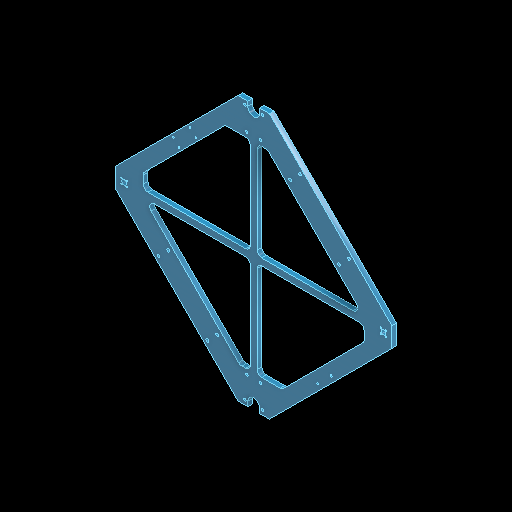
# Autodesk Inventor part: z_plate
Saved by Autodesk Inventor 2026.1 (Build 301233000, 233)
## iProperties
Created: 2025-09-21
Part Number: z_plate
Material: Aluminum 6061
Document SubType Name: Modeling
Designer: drago
Density: 2.7 g/cm^3
Appearance: Sky Blue Dark
Mass: 2273.65 g
Surface Area: 2214.69 cm^2
Volume: 842.092 cm^3
Author: drago
Autodesk Inventor part; units mm, degrees
ref_plane "YZ Plane" through (0, 0, 0) normal (1, 0, 0) x (0, 1, 0)
ref_plane "XZ Plane" through (0, 0, 0) normal (0, 1, 0) x (-1, 0, 0)
sketch "Sketch2" plane through (0, 0, 0) normal (0, 0, 1) x (1, 0, 0)
  circle A0 centre (0, 277.5) radius 8 construction
  circle A1 centre (0, 277.5) radius 13
  circle A2 centre (0, 277.5) radius 10.5 construction
  line L0 (25, 287.5) -> (-25, 287.5) construction
  line L1 (-25, 287.5) -> (-25, 222.5) construction
  line L2 (-25, 222.5) -> (25, 222.5) construction
  line L3 (25, 222.5) -> (25, 287.5) construction
  circle A3 centre (15, 228.5) radius 2.7
  circle A4 centre (-15, 228.5) radius 2.7
  circle A5 centre (-19, 277.5) radius 2.7
  circle A6 centre (19, 277.5) radius 2.7
  circle A7 centre (0, -277.5) radius 8 construction
  circle A8 centre (0, -277.5) radius 13
  circle A9 centre (0, -277.5) radius 10.5 construction
  line L4 (25, -287.5) -> (-25, -287.5) construction
  line L5 (-25, -287.5) -> (-25, -222.5) construction
  line L6 (-25, -222.5) -> (25, -222.5) construction
  line L7 (25, -222.5) -> (25, -287.5) construction
  circle A10 centre (-15, -228.5) radius 2.7
  circle A11 centre (15, -228.5) radius 2.7
  circle A12 centre (-19, -277.5) radius 2.7
  circle A13 centre (19, -277.5) radius 2.7
  line L8 (10.5, -277.5) -> (10.5, -287.5) construction
  line L9 (-10.5, -277.5) -> (-10.5, -287.5) construction
  line L10 (10.5, 277.5) -> (10.5, 287.5) construction
  line L11 (-10.5, 277.5) -> (-10.5, 287.5) construction
  circle A14 centre (281.7, 0) radius 5.25
  circle A15 centre (-281.7, 0) radius 5.25
  line L12 (0, -321.7336) -> (321.7336, 0)
  line L13 (321.7336, 0) -> (0, 321.7336)
  line L14 (0, 321.7336) -> (-321.7336, 0)
  line L15 (-321.7336, 0) -> (0, -321.7336)
  line L16 (321.7336, 0) -> (-321.7336, 0) construction
  line L17 (0, -321.7336) -> (455, -321.7336) construction
  line L18 (300.5, 21.2336) -> (300.5, -21.2336)
  line L19 (-300.5, 21.2336) -> (-300.5, -21.2336)
  line L20 (-24.2336, 297.5) -> (24.2336, 297.5) construction
  line L21 (-34.2336, 287.5) -> (34.2336, 287.5)
  line L22 (-24.2336, -297.5) -> (24.2336, -297.5) construction
  line L23 (-34.2336, -287.5) -> (34.2336, -287.5)
  line L24 (-9.5, 297.5) -> (-3.976, 284.442) construction
  line L25 (9.5, 297.5) -> (3.976, 284.442) construction
  line L26 (-14.929, 297.5) -> (-9.9883, 285.8207)
  line L27 (14.929, 297.5) -> (9.9883, 285.8207)
  line L28 (-9.5, -297.5) -> (-3.976, -284.442) construction
  line L29 (9.5, -297.5) -> (3.976, -284.442) construction
  line L30 (14.929, -297.5) -> (9.9883, -285.8207)
  line L31 (-14.929, -297.5) -> (-9.9883, -285.8207)
  line L32 (13, 277.5) -> (13, 287.5)
  line L33 (-13, 277.5) -> (-13, 287.5)
  line L34 (-13, -277.5) -> (-13, -287.5)
  line L35 (13, -277.5) -> (13, -287.5)
  line L36 (281.7, 0) -> (287.3569, 5.6569) construction
  line L37 (281.7, 0) -> (289.7, 0) construction
  circle A16 centre (287.3569, 5.6569) radius 1.6
  circle A17 centre (276.0431, 5.6569) radius 1.6
  circle A18 centre (276.0431, -5.6569) radius 1.6
  circle A19 centre (287.3569, -5.6569) radius 1.6
  line L38 (-281.7, 0) -> (-287.3569, 5.6569) construction
  circle A20 centre (-287.3569, 5.6569) radius 1.6
  circle A21 centre (-287.3569, -5.6569) radius 1.6
  circle A22 centre (-276.0431, -5.6569) radius 1.6
  circle A23 centre (-276.0431, 5.6569) radius 1.6
  line L39 (0, -321.7336) -> (0, 321.7336) construction
  point P0 (0, 0)
  point P1 (-10.6987, -287.5)
  point P2 (10.6987, -287.5)
  point P3 (10.6987, 287.5)
  point P4 (-10.6987, 287.5)
  point P5 (300.5, 292.5)
  point P6 (300.5, -292.5)
  point P7 (-300.5, -292.5)
  point P8 (-300.5, 292.5)
  dimension "d256" = 16
  dimension "d258" = 277.5
  dimension "d259" = 26
  dimension "d260" = 21
  dimension "d262" = 10
  dimension "d263" = 65
  dimension "d271" = 6
  dimension "d272" = 10
  dimension "d275" = 6
  dimension "d276" = 10
  dimension "d285" = 10
  dimension "d300" = 10.5
  dimension "d302" = 281.7
  dimension "d321" = 45
  dimension "d322" = 455
  dimension "d323" = 18.8
  dimension "d325" = 20
  dimension "d330" = 67.07
  dimension "d331" = 9.5
  dimension "d336" = 14.929
  dimension "d391" = 8
  dimension "d392" = 45
  dimension "d394" = 3.2
  dimension "d397" = 360
  dimension "d399" = 8
  dimension "d400" = 45
  dimension "d404" = 360
  dimension "d432" = 5.4
  dimension "d433" = 50
  dimension "d483" = 10
  constraints: 80 end point, 34 point on line, 24 centre point, 16 point on circle, 12 equal radius, 9 perpendicular, 8 equal length, 8 symmetric about line, 7 horizontal, 6 coincident, 6 parallel, 6 tangent, 5 vertical, 2 midpoint, 27 other
  measures "d256" diameter of A0
  measures "d258" distance of point (0, 0) A0.centre
  measures "d259" diameter of A1
  measures "d260" diameter of A2
  measures "d262" distance from line of A2.centre L0
  measures "d263" distance of L0.end L1.end
  measures "d271" distance from line of L2 A3.centre
  measures "d272" distance from line of L3 A3.centre
  measures "d275" distance from line of L3 A6.centre
  measures "d276" distance from line of L0 A6.centre
  measures "d285" distance from line of L4 A8.centre
  measures "d300" diameter of A14
  measures "d302" distance of point (0, 0) L36.start
  measures "d321" angle of L17 L12
  measures "d322" distance of L13.end L12.end
  measures "d323" distance from line of L18 L36.start
  measures "d325" distance from line of A1.centre L20
  measures "d330" angle of L25 L20
  measures "d331" horizontal distance of A1.centre L25.start
  measures "d336" horizontal distance of A1.centre L27.start
  measures "d391" distance of L36.start L36.end
  measures "d392" angle of L37 L36
  measures "d394" diameter of A16
  measures "d399" distance of L38.start L38.end
  measures "d400" angle of L16 L38
  measures "d432" diameter of A3
  measures "d433" distance of L1.end L2.end
  measures "d483" distance from line of A1.centre L21
ref_plane "Work Plane1" through (0, 0, 0) normal (0, 0, 1) x (1, 0, 0)
sketch "Sketch3" plane through (0, 0, 0) normal (0, 0, 1) x (1, 0, 0)
  line L0 (-160.8668, -160.8668) -> (160.8668, 160.8668) construction
  line L1 (-160.8668, -160.8668) -> (294.1332, -160.8668) construction
  line L2 (279.5102, 35.1523) -> (35.1523, 279.5102) construction
  line L3 (35.1523, 279.5102) -> (6.8681, 251.2259) construction
  line L4 (6.8681, 251.2259) -> (251.2259, 6.8681) construction
  line L5 (251.2259, 6.8681) -> (279.5102, 35.1523) construction
  circle A0 centre (19, 277.5) radius 2.7 projected
  circle A1 centre (15, 228.5) radius 2.7 projected
  line L6 (-35.1523, -279.5102) -> (-279.5102, -35.1523) construction
  line L7 (-279.5102, -35.1523) -> (-251.2259, -6.8681) construction
  line L8 (-251.2259, -6.8681) -> (-6.8681, -251.2259) construction
  line L9 (-6.8681, -251.2259) -> (-35.1523, -279.5102) construction
  circle A2 centre (-79.5495, -185.6155) radius 3.1
  circle A3 centre (-100.7627, -206.8287) radius 3.1
  circle A4 centre (-185.6155, -79.5495) radius 3.1
  circle A5 centre (-206.8287, -100.7627) radius 3.1
  line L10 (-160.8668, 160.8668) -> (160.8668, -160.8668) construction
  circle A6 centre (206.8287, 100.7627) radius 3.1
  circle A7 centre (185.6155, 79.5495) radius 3.1
  circle A8 centre (100.7627, 206.8287) radius 3.1
  circle A9 centre (79.5495, 185.6155) radius 3.1
  line L11 (-175.0089, 138.2394) -> (-138.2394, 175.0089) construction
  line L12 (-138.2394, 175.0089) -> (-125.5115, 162.281) construction
  line L13 (-125.5115, 162.281) -> (-162.281, 125.5115) construction
  line L14 (-162.281, 125.5115) -> (-175.0089, 138.2394) construction
  circle A10 centre (-138.2394, 175.0089) radius 2.1
  circle A11 centre (-125.5115, 162.281) radius 2.1
  circle A12 centre (-162.281, 125.5115) radius 2.1
  circle A13 centre (-175.0089, 138.2394) radius 2.1
  line L15 (-162.281, 125.5115) -> (-138.2394, 175.0089) construction
  line L16 (-175.0089, 138.2394) -> (-125.5115, 162.281) construction
  line L17 (138.9465, -168.645) -> (168.645, -138.9465) construction
  circle A14 centre (168.645, -138.9465) radius 2.1
  circle A15 centre (138.9465, -168.645) radius 2.1
  line L18 (21.0102, 265.3681) -> (265.3681, 21.0102) construction
  line L19 (-265.3681, -21.0102) -> (-21.0102, -265.3681) construction
  point P0 (0, 0)
  point P1 (-150.2602, 150.2602)
  point P2 (153.7957, -153.7957)
  dimension "d349" = 455
  dimension "d350" = 45
  dimension "d353" = 40
  dimension "d354" = 10
  dimension "d362" = 75
  dimension "d363" = 5
  dimension "d365" = 5
  dimension "d366" = 75
  dimension "d370" = 5
  dimension "d371" = 75
  dimension "d373" = 5
  dimension "d374" = 75
  dimension "d436" = 52
  dimension "d437" = 18
  dimension "d438" = 221.5
  dimension "d439" = 4.2
  dimension "d440" = 42
  dimension "d442" = 217.5
  dimension "d450" = 6.2
  dimension "d482" = 405
  constraints: 40 end point, 14 centre point, 9 midpoint, 8 equal radius, 7 perpendicular, 6 coincident, 6 parallel, 4 symmetric about line, 3 equal length, 2 point on line, 1 collinear, 1 horizontal, 11 other
  measures "d349" distance of L0.start L0.end
  measures "d350" angle of L1 L0
  measures "d353" distance of L3.end L2.end
  measures "d354" distance from line of L3 A0.centre
  measures "d362" distance from line of L0 A2.centre
  measures "d363" distance from line of L8 A2.centre
  measures "d365" distance from line of L6 A3.centre
  measures "d366" distance from line of L0 A3.centre
  measures "d370" distance from line of L2 A6.centre
  measures "d371" distance from line of L0 A6.centre
  measures "d373" distance from line of L4 A7.centre
  measures "d374" distance from line of L0 A7.centre
  measures "d436" distance of L11.start L11.end
  measures "d437" distance of L11.end L12.end
  measures "d438" distance from line of point (0, 0) L11
  measures "d439" diameter of A10
  measures "d440" distance of L17.start L17.end
  measures "d442" distance from line of point (0, 0) L17
  measures "d450" diameter of A6
  measures "d482" distance between parallel lines of L19 L18
extrude "Extrusion12" add sketch "Sketch2" against normal blind 10 contours L32 L21 L13 L18 L12 L23 L35 A8 L34 L15 L19 L14 L33 A1
hole "Hole2" at (100.7627, 206.8287, 0) at (79.5495, 185.6155, 0) at (206.8287, 100.7627, 0) at (185.6155, 79.5495, 0) at (-79.5495, -185.6155, 0) at (-100.7627, -206.8287, 0) at (-185.6155, -79.5495, 0) at (-206.8287, -100.7627, 0) direction (0, 0, -1) diameter 6.2 end through all
hole "Hole4" at (-175.0089, 138.2394, 0) at (-162.281, 125.5115, 0) at (-125.5115, 162.281, 0) at (-138.2394, 175.0089, 0) at (168.645, -138.9465, 0) at (138.9465, -168.645, 0) direction (0, 0, -1) diameter 4.2 end through all
sketch "Sketch5" plane through (0, 0, 0) normal (0, 0, 1) x (1, 0, 0)
  line L0 (29.9874, 217.5) -> (-61.8072, 217.5)
  line L1 (139.6536, -139.6536) -> (-139.6536, 139.6536) construction
  line L2 (-29.9874, -217.5) -> (-263.3973, 15.9099)
  line L3 (61.8072, -217.5) -> (-29.9874, -217.5)
  line L4 (247.4874, 0) -> (-247.4874, 0) construction
  line L5 (-61.8072, 217.5) -> (-263.3973, 15.9099)
  line L6 (61.8072, -217.5) -> (263.3973, -15.9099)
  line L7 (0, -217.5) -> (0, 217.5) construction
  line L8 (263.3973, -15.9099) -> (29.9874, 217.5)
  line L9 (-123.7437, -123.7437) -> (123.7437, 123.7437) construction
  line L10 (-217.5, 61.8072) -> (-217.5, -29.9874)
  line L11 (217.5, 29.9874) -> (217.5, -61.8072)
  line L12 (-247.4874, 0) -> (-29.9874, 217.5)
  line L13 (247.4874, 0) -> (29.9874, -217.5)
  line L14 (-7.5, 217.5) -> (-7.5, -217.5)
  line L15 (7.5, 217.5) -> (7.5, -217.5)
  line L16 (-239.9874, 7.5) -> (239.9874, 7.5)
  line L17 (239.9874, -7.5) -> (-239.9874, -7.5)
  line L18 (-239.9874, -7.5) -> (-239.9874, 39.3198)
  line L19 (239.9874, 7.5) -> (239.9874, -39.3198)
  point P0 (0, 0)
  point P1 (-7.5, -7.5)
  point P2 (7.5, -7.5)
  point P3 (-7.5, 7.5)
  point P4 (7.5, 7.5)
  point P5 (217.5, -29.9874)
  point P6 (-217.5, 29.9874)
  dimension "d460" = 197.5
  dimension "d461" = 197.5
  dimension "d465" = 175
  dimension "d466" = 217.5
  dimension "d467" = 45
  dimension "d468" = 217.5
  dimension "d469" = 175
  dimension "d473" = 15
  dimension "d475" = 15
  constraints: 40 end point, 22 point on line, 8 perpendicular, 4 midpoint, 3 horizontal, 3 vertical, 2 parallel, 7 other
  measures "d460" distance from line of point (0, 0) L5
  measures "d461" distance from line of L6 point (0, 0)
  measures "d465" distance from line of point (0, 0) L8
  measures "d466" distance from line of point (0, 0) L0
  measures "d467" angle of L7 L1
  measures "d468" distance from line of point (0, 0) L10
  measures "d469" distance from line of point (0, 0) L12
  measures "d473" distance between parallel lines of L15 L14
  measures "d475" distance between parallel lines of L17 L16
extrude "Extrusion15" cut sketch "Sketch5" against normal blind 217.5 contours L8 L11 L16 L15 L0 | L8 L16 L11 | L14 L16 L10 L12 L0 | L12 L10 L5 L0 | L17 L11 L13 L3 L15 | L19 L6 L11 L13 | L13 L11 L17 | L12 L18 L5 L10 | L10 L16 L12 | L14 L3 L2 L10 L17 | L11 L6 L3 L13 | L10 L2 L17
fillet "Fillet2" radius 10 18 edges at (-61.8072, 217.5, -5) (29.9874, 217.5, -5) (-7.5, 217.5, -5) (239.9874, -7.5, -5) (-7.5, -7.5, -5) (239.9874, -39.3198, -5) (61.8072, -217.5, -5) (-7.5, -217.5, -5) (-7.5, 7.5, -5) (-29.9874, -217.5, -5) (7.5, 7.5, -5) (-239.9874, 7.5, -5) (-239.9874, 39.3198, -5) (7.5, -7.5, -5) (7.5, 217.5, -5) (7.5, -217.5, -5) (239.9874, 7.5, -5) (-239.9874, -7.5, -5)
equation "\"dist_rails\" = 555"
equation "\"dist_leadscrews\" = 563.4"
equation "\"diam_leadscrew_hole\" = 10.5"
equation "\"z_plate_width\" = 455"
equation "\"delta\" = 5"
equation "\"rail_angle\" = 67.07deg"
equation "\"rail_D\" = 9.5"
equation "\"rail_diam\" = 16"
equation "\"rail_dist\" = 405"
body "Solid10"
